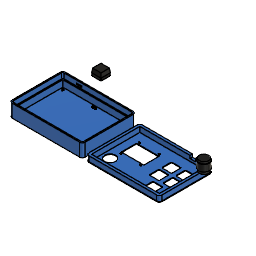
Placa (Autodesk Fusion 360 design; units mm, degrees)
Autodesk Fusion 360 part; units mm, degrees
note: some values were not read from the file. Chosen so that the rebuilt part matches the saved one: which bodies a step acts on. Set by a fixed rule: which sketch regions a step uses.
sketch "Boceto1" plane through (0, 0, 0) normal (0, 0, 1) x (1, 0, 0)
  line L0 (-2, 76) -> (102, 76)
  line L1 (106, 72) -> (106, -2)
  line L2 (102, -6) -> (-2, -6)
  line L3 (-6, -2) -> (-6, 72)
  arc A0 (102, -6) -> (106, -2) centre (102, -2) ccw
  arc A1 (106, 72) -> (102, 76) centre (102, 72) ccw
  arc A2 (-2, 76) -> (-6, 72) centre (-2, 72) ccw
  arc A3 (-6, -2) -> (-2, -6) centre (-2, -2) ccw
  line L4 (-2, 72) -> (102, 72)
  line L5 (-2, -2) -> (-2, 72)
  line L6 (102, -2) -> (-2, -2)
  line L7 (102, 72) -> (102, -2)
  line L8 (0, 0) -> (100, 0)
  line L9 (100, 0) -> (100, 70)
  line L10 (100, 70) -> (0, 70)
  line L11 (0, 70) -> (0, 0)
  circle A4 centre (1.8, 68) radius 1
  circle A5 centre (1.8, 68) radius 1.5
  circle A6 centre (1.8, 2) radius 1
  circle A7 centre (48.2, 68) radius 1
  circle A8 centre (48.2, 68) radius 1.5
  circle A9 centre (1.8, 2) radius 1.5
  circle A10 centre (48.2, 2) radius 1.5
  circle A11 centre (48.2, 2) radius 1
  circle A12 centre (98.2, 2) radius 1.5
  circle A13 centre (98.2, 2) radius 1
  circle A14 centre (51.8, 2) radius 1
  circle A15 centre (51.8, 2) radius 1.5
  circle A16 centre (51.8, 68) radius 1.5
  circle A17 centre (51.8, 68) radius 1
  circle A18 centre (98.2, 68) radius 1
  circle A19 centre (98.2, 68) radius 1.5
  arc A20 (-2, 74) -> (-4, 72) centre (-2, 72) ccw
  line L12 (-4, -2) -> (-4, 72)
  arc A21 (-4, -2) -> (-2, -4) centre (-2, -2) ccw
  line L13 (102, -4) -> (-2, -4)
  arc A22 (102, -4) -> (104, -2) centre (102, -2) ccw
  line L14 (104, 72) -> (104, -2)
  arc A23 (104, 72) -> (102, 74) centre (102, 72) ccw
  line L15 (-2, 74) -> (102, 74)
  point P0 (-6, 76)
  point P1 (106, 76)
  point P2 (-6, -6)
  point P3 (22.5, -6)
  point P4 (50, 70)
  point P5 (50, 70)
  dimension "d29" = 4
  dimension "d30" = 4
  dimension "d31" = 4
  dimension "d32" = 4
  dimension "d35" = 4
  dimension "d285" = 100
  dimension "d286" = 70
  dimension "d287" = 2
  dimension "d288" = 0.5
  dimension "d289" = 2
  dimension "d290" = 66
  dimension "d291" = 2
  dimension "d292" = 46.4
  dimension "d293" = 2
  dimension "d294" = 1.8
  dimension "d295" = 0.5
  dimension "d296" = 0.5
  dimension "d297" = 2
  dimension "d298" = 1.8
  dimension "d303" = 2
  dimension "d306" = 50
  dimension "d307" = 0
  dimension "d308" = 1.8
  dimension "d321" = 2
  dimension "d322" = 2
  dimension "d323" = -2
  constraint horizontal L0
  constraint vertical L1
  constraint horizontal L2
  constraint vertical L3
  constraint tangent L1 A0
  constraint tangent L2 A0
  constraint coincident P1 L0
  constraint coincident P1 L1
  constraint tangent L0 A1
  constraint tangent L1 A1
  constraint coincident P0 L0
  constraint coincident P0 L3
  constraint tangent L0 A2
  constraint tangent L3 A2
  constraint coincident P2 L2
  constraint coincident P2 L3
  constraint tangent L2 A3
  constraint tangent L3 A3
  constraint coincident L2 P3
  constraint horizontal L8
  constraint vertical L9
  constraint horizontal L10
  constraint vertical L11
  constraint coincident L8.start L11.end
  constraint midpoint L10 P5
  measures "d29" radius of A0
  measures "d30" radius of A1
  measures "d31" radius of A2
  measures "d32" radius of A3
  measures "d285" distance of L8.start L8.end
  measures "d286" distance of L8.start L10.end
  measures "d287" diameter of A4
  measures "d289" diameter of A6
  measures "d290" vertical distance of A4.centre A6.centre
  measures "d291" diameter of A7
  measures "d292" horizontal distance of A4.centre A7.centre
  measures "d293" distance of L10 A4.centre
  measures "d294" distance of L11 A4.centre
  measures "d297" distance of L8 A6.centre
  measures "d298" horizontal distance of A7.centre P5
  measures "d303" distance of L10 A7.centre
  measures "d308" distance of L11 A6.centre
  measures "d321" distance of L5 L11
  measures "d322" distance of L4 L10
extrude "Extruir10" add sketch "Boceto1" along normal blind 2 contours L8 L9 L10 L11 | A4 | A5 | A6 | A7 | A8 | A9 | A10 | A11 | A12 | A13 | A14 | A15 | A16 | A17 | A18 | A19 makes body 1
extrude "Extruir41" add sketch "Boceto1" along normal blind 3 separate body contours A5 makes body 2
extrude "Extruir42" add sketch "Boceto1" along normal blind 4 contours A4 bodies 2
pattern_linear "Patrón R4" count 2 spacing 66 along (0, -1, 0) count 2 spacing 46.4 along (1, 0, 0) of bodies 2 makes body 3 at (3.2981, 1.9252, 2) makes body 4 at (49.5822, 68.5827, 2) makes body 5 at (48.6063, 3.4439, 2)
pattern_linear "Patrón R5" count 2 spacing 50 along (1, 0, 0) of bodies 2 3 4 5 makes body 6 at (53.1822, 68.5827, 2) makes body 7 at (51.1157, 0.6652, 2) makes body 8 at (99.5822, 68.5827, 2) makes body 9 at (99.6981, 1.9252, 2)
combine "Combinar3" operation add target body 1 tool bodies 6 3 4 5 7 9 8 2
extrude "Extruir13" add sketch "Boceto1" along normal blind 2 contours L4 L5 L6 L7 bodies 1
extrude "Extruir14" add sketch "Boceto1" along normal blind 20 contours L0 L1 L2 L3 A0 A1 A2 A3 | A20 L12 A21 L13 A22 L14 A23 L15 bodies 1
sketch "Boceto3" plane through (0, 76, 0) normal (0, 1, 0) x (-1, 0, 0)
  line L0 (-102, 0) -> (2, 0)
  line L1 (2, 0) -> (2, 20)
  line L2 (2, 20) -> (-102, 20)
  line L3 (-102, 20) -> (-102, 0)
  line L4 (-25.1, 16) -> (-17, 16)
  line L5 (-23.55, 13) -> (-18.55, 13)
  line L6 (-25.1, 16) -> (-25.1, 14.7)
  line L7 (-17, 16) -> (-17, 14.7)
  line L8 (-17, 14.7) -> (-18.55, 13)
  line L9 (-25.1, 14.7) -> (-23.55, 13)
  line L10 (2, 0) -> (-102, 0)
  dimension "d97" = 8.1
  dimension "d98" = 5
  dimension "d99" = 3
  dimension "d101" = 1.3
  dimension "d102" = 1.3
  dimension "d103" = 19
  dimension "d105" = 16
  constraint horizontal L4
  constraint horizontal L5
  constraint perpendicular L4 L6
  constraint vertical L7
  measures "d97" distance of L4.start L4.end
  measures "d98" distance of L5.start L5.end
  measures "d99" distance of L4 L5
  measures "d101" distance of L4.start L6.end
  measures "d102" distance of L4.end L7.end
  measures "d103" distance of L1 L7
  measures "d105" distance of L4 L10
extrude "Extruir15" cut sketch "Boceto3" against normal blind 18 contours L4 L5 L6 L7 L8 L9 bodies 1
sketch "Boceto4" plane through (0, 0, 20) normal (0, 0, 1) x (-1, 0, 0)
  line L0 (2, -72) -> (-102, -72)
  line L1 (-102, -72) -> (-102, 2)
  line L2 (-102, 2) -> (2, 2)
  line L3 (2, 2) -> (2, -72)
  arc A0 (2, -76) -> (6, -72) centre (2, -72) ccw
  line L4 (6, -72) -> (6, 2)
  arc A1 (6, 2) -> (2, 6) centre (2, 2) ccw
  line L5 (2, 6) -> (-102, 6)
  arc A2 (-102, 6) -> (-106, 2) centre (-102, 2) ccw
  line L6 (-106, 2) -> (-106, -72)
  arc A3 (-106, -72) -> (-102, -76) centre (-102, -72) ccw
  line L7 (-102, -76) -> (2, -76)
  line L8 (2, 5.9687) -> (-102, 5.9687)
  arc A4 (-102, 5.9687) -> (-105.9688, 2) centre (-102, 2) ccw
  line L9 (-105.9688, 2) -> (-105.9688, -72)
  arc A5 (-105.9688, -72) -> (-102, -75.9688) centre (-102, -72) ccw
  line L10 (-102, -75.9688) -> (2, -75.9688)
  arc A6 (2, -75.9688) -> (5.9688, -72) centre (2, -72) ccw
  line L11 (5.9687, -72) -> (5.9687, 2)
  arc A7 (5.9687, 2) -> (2, 5.9688) centre (2, 2) ccw
  line L12 (2, 3.9687) -> (-102, 3.9687)
  arc A8 (-102, 3.9687) -> (-103.9688, 2) centre (-102, 2) ccw
  line L13 (-103.9688, 2) -> (-103.9688, -72)
  arc A9 (-103.9688, -72) -> (-102, -73.9688) centre (-102, -72) ccw
  line L14 (-102, -73.9688) -> (2, -73.9687)
  arc A10 (2, -73.9687) -> (3.9687, -72) centre (2, -72) ccw
  line L15 (3.9687, -72) -> (3.9688, 2)
  arc A11 (3.9688, 2) -> (2, 3.9688) centre (2, 2) ccw
  dimension "d328" = -2
extrude "Extruir16" cut sketch "Boceto4" against normal blind 8 contours L12 A8 L13 A9 L14 A10 L15 A11 bodies 1
extrude "Extruir17" add sketch "Boceto4" along normal blind 8 separate body contours L8 A4 L9 A5 L10 A6 L11 A7 | L12 A8 L13 A9 L14 A10 L15 A11 makes body 10
extrude "Extruir18" add sketch "Boceto4" along normal blind 9 contours A0 L4 A1 L5 A2 L6 A3 L7 bodies 10
extrude "Extruir19" cut sketch "Boceto4" along normal blind 8 contours A0 L4 A1 L5 A2 L6 A3 L7 bodies 10
extrude "Extruir20" add 1 faces at (32.6667, 73.3229, 28) along direction (0, 0, 1) blind 1 on bodies 10 bodies 10
extrude "Extruir21" add sketch "Boceto4" along normal blind 9 contours L0 L1 L2 L3 bodies 10
extrude "Extruir22" cut sketch "Boceto4" along normal blind 8 contours L0 L1 L2 L3 bodies 10
move_body "Desplazar1" bodies 10 to x (1, 0, 0) y (0, 1, 0) z (0, 0, 1) at (115, 0, 0)
sketch "Boceto5" plane through (0, 0, 29) normal (0, 0, 1) x (-1, 0, 0)
  line L0 (-217, -76) -> (-113, -76)
  arc A0 (-113, -76) -> (-109, -72) centre (-113, -72) ccw
  line L1 (-109, -72) -> (-109, 2)
  arc A1 (-109, 2) -> (-113, 6) centre (-113, 2) ccw
  line L2 (-113, 6) -> (-217, 6)
  arc A2 (-217, 6) -> (-221, 2) centre (-217, 2) ccw
  line L3 (-221, 2) -> (-221, -72)
  arc A3 (-221, -72) -> (-217, -76) centre (-217, -72) ccw
  line L4 (-170.1727, -59.9244) -> (-205.5227, -59.9244)
  line L5 (-205.5227, -59.9244) -> (-205.5227, -26.5744)
  line L6 (-205.5227, -26.5744) -> (-170.1727, -26.5744)
  line L7 (-170.1727, -26.5744) -> (-170.1727, -59.9244)
  circle A4 centre (-172.6727, -57.4244) radius 1.25
  line L8 (-187.8477, -59.9244) -> (-187.8477, -26.5744)
  circle A5 centre (-203.0227, -57.4244) radius 1.25
  line L9 (-170.1727, -43.2494) -> (-205.5227, -43.2494)
  circle A6 centre (-172.6727, -29.0744) radius 1.25
  circle A7 centre (-203.0227, -29.0744) radius 1.25
  line L10 (-170.6477, -54.9244) -> (-205.0477, -54.9244)
  line L11 (-205.0477, -54.9244) -> (-205.0477, -31.9244)
  line L12 (-205.0477, -31.9244) -> (-170.6477, -31.9244)
  line L13 (-170.6477, -31.9244) -> (-170.6477, -54.9244)
  circle A8 centre (-205.4274, -14.9454) radius 7.2
  circle A9 centre (-205.4274, -14.9454) radius 8.2
  line L14 (-118, -57) -> (-131, -57)
  line L15 (-132, -56) -> (-132, -43)
  line L16 (-131, -42) -> (-118, -42)
  line L17 (-117, -43) -> (-117, -56)
  arc A10 (-118, -57) -> (-117, -56) centre (-118, -56) ccw
  arc A11 (-132, -56) -> (-131, -57) centre (-131, -56) ccw
  arc A12 (-131, -42) -> (-132, -43) centre (-131, -43) ccw
  arc A13 (-117, -43) -> (-118, -42) centre (-118, -43) ccw
  arc A14 (-153.4221, -56) -> (-152.4221, -57) centre (-152.4221, -56) ccw
  line L18 (-153.4221, -56) -> (-153.4221, -43)
  arc A15 (-152.4221, -42) -> (-153.4221, -43) centre (-152.4221, -43) ccw
  line L19 (-152.4221, -42) -> (-139.4221, -42)
  arc A16 (-138.4221, -43) -> (-139.4221, -42) centre (-139.4221, -43) ccw
  line L20 (-138.4221, -43) -> (-138.4221, -56)
  arc A17 (-139.4221, -57) -> (-138.4221, -56) centre (-139.4221, -56) ccw
  line L21 (-139.4221, -57) -> (-152.4221, -57)
  arc A18 (-132.0698, -36.5317) -> (-131.0698, -37.5317) centre (-131.0698, -36.5317) ccw
  line L22 (-132.0698, -36.5317) -> (-132.0698, -23.5317)
  arc A19 (-131.0698, -22.5317) -> (-132.0698, -23.5317) centre (-131.0698, -23.5317) ccw
  line L23 (-131.0698, -22.5317) -> (-118.0698, -22.5317)
  arc A20 (-117.0698, -23.5317) -> (-118.0698, -22.5317) centre (-118.0698, -23.5317) ccw
  line L24 (-117.0698, -23.5317) -> (-117.0698, -36.5317)
  arc A21 (-118.0698, -37.5317) -> (-117.0698, -36.5317) centre (-118.0698, -36.5317) ccw
  line L25 (-118.0698, -37.5317) -> (-131.0698, -37.5317)
  arc A22 (-153.4221, -36.8108) -> (-152.4221, -37.8108) centre (-152.4221, -36.8108) ccw
  line L26 (-153.4221, -36.8108) -> (-153.4221, -23.8108)
  arc A23 (-152.4221, -22.8108) -> (-153.4221, -23.8108) centre (-152.4221, -23.8108) ccw
  line L27 (-152.4221, -22.8108) -> (-139.4221, -22.8108)
  arc A24 (-138.4221, -23.8108) -> (-139.4221, -22.8108) centre (-139.4221, -23.8108) ccw
  line L28 (-138.4221, -23.8108) -> (-138.4221, -36.8108)
  arc A25 (-139.4221, -37.8108) -> (-138.4221, -36.8108) centre (-139.4221, -36.8108) ccw
  line L29 (-139.4221, -37.8108) -> (-152.4221, -37.8108)
  arc A26 (-141.9784, -16.2261) -> (-140.9784, -17.2261) centre (-140.9784, -16.2261) ccw
  line L30 (-141.9784, -16.2261) -> (-141.9784, -3.2261)
  arc A27 (-140.9784, -2.2261) -> (-141.9784, -3.2261) centre (-140.9784, -3.2261) ccw
  line L31 (-140.9784, -2.2261) -> (-127.9784, -2.2261)
  arc A28 (-126.9784, -3.2261) -> (-127.9784, -2.2261) centre (-127.9784, -3.2261) ccw
  line L32 (-126.9784, -3.2261) -> (-126.9784, -16.2261)
  arc A29 (-127.9784, -17.2261) -> (-126.9784, -16.2261) centre (-127.9784, -16.2261) ccw
  line L33 (-127.9784, -17.2261) -> (-140.9784, -17.2261)
  point P0 (-108.3558, -46.4242)
  point P1 (-117, -57)
  point P2 (-132, -57)
  point P3 (-117, -42)
  dimension "d125" = 35.35
  dimension "d126" = 33.35
  dimension "d127" = 2.5
  dimension "d131" = 2.5
  dimension "d132" = 2.5
  dimension "d133" = 34.4
  dimension "d134" = 23
  dimension "d135" = 2.5
  dimension "d136" = 0.475
  dimension "d141" = 14.4
  dimension "d142" = 1
  dimension "d256" = 15
  dimension "d257" = 15
  dimension "d258" = 1
  dimension "d259" = 1
  dimension "d260" = 1
  dimension "d261" = 1
  dimension "d262" = 1
  constraint horizontal L4
  constraint vertical L5
  constraint horizontal L6
  constraint vertical L7
  constraint midpoint L4 L8.start
  constraint midpoint L6 L8.end
  constraint symmetric A4 L8 A5
  constraint midpoint L7 L9.start
  constraint midpoint L5 L9.end
  constraint symmetric A4 L9 A6
  constraint symmetric A5 L9 A7
  constraint horizontal L10
  constraint vertical L11
  constraint horizontal L12
  constraint vertical L13
  constraint horizontal L14
  constraint vertical L15
  constraint horizontal L16
  constraint vertical L17
  constraint coincident P1 L14
  constraint coincident P1 L17
  constraint tangent L14 A10
  constraint tangent L17 A10
  constraint coincident P2 L14
  constraint coincident P2 L15
  constraint tangent L14 A11
  constraint tangent L15 A11
  constraint equal A10 A11
  constraint tangent L15 A12
  constraint tangent L16 A12
  constraint equal A10 A12
  constraint coincident P3 L16
  constraint coincident P3 L17
  constraint tangent L16 A13
  constraint tangent L17 A13
  constraint equal A10 A13
  constraint horizontal L21
  constraint vertical L18
  constraint horizontal L19
  constraint vertical L20
  constraint tangent A17 L21
  constraint tangent L20 A17
  constraint tangent A14 L21
  constraint tangent A14 L18
  constraint equal A14 A17
  constraint tangent L18 A15
  constraint tangent A15 L19
  constraint equal A15 A17
  constraint tangent L19 A16
  constraint tangent A16 L20
  constraint equal A16 A17
  constraint horizontal L25
  constraint vertical L22
  constraint horizontal L23
  constraint vertical L24
  constraint tangent A21 L25
  constraint tangent L24 A21
  constraint tangent A18 L25
  constraint tangent A18 L22
  constraint equal A18 A21
  constraint tangent L22 A19
  constraint tangent A19 L23
  constraint equal A19 A21
  constraint tangent L23 A20
  constraint tangent A20 L24
  constraint equal A20 A21
  constraint horizontal L29
  constraint vertical L26
  constraint horizontal L27
  constraint vertical L28
  constraint tangent A25 L29
  constraint tangent L28 A25
  constraint tangent A22 L29
  constraint tangent A22 L26
  constraint equal A22 A25
  constraint tangent L26 A23
  constraint tangent A23 L27
  constraint equal A23 A25
  constraint tangent L27 A24
  constraint tangent A24 L28
  constraint equal A24 A25
  constraint horizontal L33
  constraint vertical L30
  constraint horizontal L31
  constraint vertical L32
  constraint tangent A29 L33
  constraint tangent L32 A29
  constraint tangent A26 L33
  constraint tangent A26 L30
  constraint equal A26 A29
  constraint tangent L30 A27
  constraint tangent A27 L31
  constraint equal A27 A29
  constraint tangent L31 A28
  constraint tangent A28 L32
  constraint equal A28 A29
  measures "d125" distance of L4.start L4.end
  measures "d126" distance of L4.start L6.end
  measures "d127" diameter of A4
  measures "d131" horizontal distance of L4.start A4.centre
  measures "d132" vertical distance of L4.start A4.centre
  measures "d133" distance of L10.start L10.end
  measures "d134" distance of L10.start L12.end
  measures "d135" distance of A4.centre L10
  measures "d136" distance of L5 L11
  measures "d141" diameter of A8
  measures "d256" distance of P1 P3
  measures "d257" distance of P1 P2
  measures "d258" radius of A10
  measures "d259" radius of A17
  measures "d260" radius of A21
  measures "d261" radius of A25
  measures "d262" radius of A29
extrude "Extruir23" cut sketch "Boceto5" against normal blind 5 contours L8 L9 L10 L11 | L8 L9 L10 L13 | L8 L9 L12 L13 | L8 L9 L11 L12 bodies 10
extrude "Extruir24" add sketch "Boceto5" against normal blind 2 contours A4 | A5 | A6 | A7 bodies 10
extrude "Extruir25" cut sketch "Boceto5" against normal blind 49 contours A8 | A9 bodies 10
extrude "Extruir26" add sketch "Boceto5" along normal blind 17 separate body contours A8 makes body 11
extrude "Extruir27" add sketch "Boceto5" along normal blind 14 separate body contours A9 makes body 12
extrude "Extruir28" cut sketch "Boceto5" along normal blind 4 contours A9 bodies 12
move_body "Desplazar2" bodies 11 12 to x (1, 0, 0) y (0, 1, 0) z (0, 0, 1) at (40.9619, 25.058, 2.4329)
combine "Combinar2" operation add target body 11 tool bodies 12
sketch "Boceto8" plane through (0, 0, 29) normal (0, 0, 1) x (1, 0, 0)
  arc A0 (-8.5, -7.5) -> (-7.5, -8.5) centre (-7.5, -7.5) ccw
  line L0 (-6.5, -6.5) -> (-6.5, 6.5)
  arc A1 (8.5, 7.5) -> (7.5, 8.5) centre (7.5, 7.5) ccw
  arc A2 (7.5, -8.5) -> (8.5, -7.5) centre (7.5, -7.5) ccw
  arc A3 (7.5, 6.5) -> (6.5, 7.5) centre (6.5, 6.5) ccw
  line L1 (-6.5, 6.5) -> (6.5, 6.5)
  line L2 (-7.5, -6.5) -> (-7.5, 6.5)
  line L3 (-7.5, 8.5) -> (7.5, 8.5)
  arc A4 (-6.5, 7.5) -> (-7.5, 6.5) centre (-6.5, 6.5) ccw
  line L4 (-8.5, -7.5) -> (-8.5, 7.5)
  line L5 (6.5, -7.5) -> (-6.5, -7.5)
  arc A5 (-7.5, 8.5) -> (-8.5, 7.5) centre (-7.5, 7.5) ccw
  circle A6 centre (0, 0) radius 1.5
  line L6 (-6.5, 7.5) -> (6.5, 7.5)
  line L7 (7.5, -8.5) -> (-7.5, -8.5)
  arc A7 (6.5, -7.5) -> (7.5, -6.5) centre (6.5, -6.5) ccw
  line L8 (8.5, 7.5) -> (8.5, -7.5)
  line L9 (6.5, 6.5) -> (6.5, -6.5)
  line L10 (7.5, 6.5) -> (7.5, -6.5)
  arc A8 (-7.5, -6.5) -> (-6.5, -7.5) centre (-6.5, -6.5) ccw
  line L11 (6.5, -6.5) -> (-6.5, -6.5)
  point P0 (7.5, 7.5)
  point P1 (-7.5, -7.5)
  point P2 (-7.5, 7.5)
  dimension "d241" = 1
  dimension "d242" = 15
  dimension "d243" = 15
  dimension "d244" = 1
  dimension "d245" = 1
  dimension "d246" = 1
  dimension "d247" = 1
  dimension "d248" = 1
  dimension "d249" = 1
  dimension "d250" = 1
  dimension "d251" = 1
  dimension "d252" = 1
  dimension "d253" = 7.5
  dimension "d254" = 7.5
  dimension "d255" = 3
  constraint horizontal L6
  constraint vertical L10
  constraint horizontal L5
  constraint vertical L2
  constraint tangent L4 A5
  constraint tangent L3 A5
  constraint tangent A0 L7
  constraint tangent A0 L4
  constraint equal A0 A5
  constraint tangent A2 L7
  constraint tangent A2 L8
  constraint equal A2 A5
  constraint tangent A1 L3
  constraint tangent A1 L8
  constraint equal A1 A5
  constraint coincident P2 L6
  constraint coincident P2 L2
  constraint tangent A4 L6
  constraint tangent L2 A4
  constraint coincident P0 L6
  constraint coincident P0 L10
  constraint tangent A3 L6
  constraint tangent A3 L10
  constraint tangent A7 L10
  constraint tangent L5 A7
  constraint coincident P1 L5
  constraint coincident P1 L2
  constraint tangent L5 A8
  constraint tangent L2 A8
  constraint coincident A6.centre origin
  measures "d242" distance of P0 P2
  measures "d243" distance of P1 P2
  measures "d244" distance of L5 L7
  measures "d245" distance of L2 L4
  measures "d246" distance of L3 L6
  measures "d247" distance of L8 L10
  measures "d248" radius of A5
  measures "d249" radius of A4
  measures "d250" radius of A3
  measures "d251" radius of A7
  measures "d252" radius of A8
  measures "d253" distance of A6.centre L2
  measures "d254" distance of A6.centre L6
  measures "d255" diameter of A6
extrude "Extruir32" add sketch "Boceto8" along normal blind 10 separate body contours L0 L1 L9 L11 | A6 makes body 13
extrude "Extruir34" add sketch "Boceto8" along normal blind 4 contours A3 L2 A4 L5 L6 A7 L10 A8 bodies 13
split "Dividir3" by plane through (0, 0, 33) normal (0, 0, 1) bodies 13 makes body 14 at (-2.1667, 2.1667, 39)
loft "Solevación1" add section 1 face at (-2.1667, 2.1667, 39) section 2 face at (6.8333, 2.1667, 33) on bodies 13 14 bodies 13 14
extrude "Extruir35" cut sketch "Boceto8" along normal blind 4 contours A6 bodies 13
move_body "Desplazar14" bodies 13 to x (1, 0, 0) y (0, 1, 0) z (0, 0, 1) at (38.8109, 89.6933, 0)
copy_body "CopiarPegarCuerpos4" bodies 13 makes body 15
copy_body "CopiarPegarCuerpos5" bodies 13 makes body 16
move_body "Desplazar15" bodies 16 to x (1, 0, 0) y (0, 1, 0) z (0, 0, 1) at (59, 0, 0)
move_body "Desplazar16" bodies 15 to x (1, 0, 0) y (0, 1, 0) z (0, 0, 1) at (27, 0, 0)
copy_body "CopiarPegarCuerpos6" bodies 15 13 makes body 17 makes body 18
move_body "Desplazar17" bodies 17 18 to x (1, 0, 0) y (0, 1, 0) z (0, 0, 1) at (16.8789, 23.4733, 0)
extrude "Extruir38" cut sketch "Boceto5" against normal blind 2 contours L14 L15 L16 L17 A10 A11 A12 A13 | A14 L18 A15 L19 A16 L20 A17 L21 | A18 L22 A19 L23 A20 L24 A21 L25 | A22 L26 A23 L27 A24 L28 A25 L29 | A26 L30 A27 L31 A28 L32 A29 L33 bodies 10
sketch "Boceto9" plane through (0, 75.9687, 0) normal (0, 1, 0) x (-1, 0, 0)
  line L0 (-217, 20) -> (-113, 20)
  line L1 (-113, 20) -> (-113, 28)
  line L2 (-113, 28) -> (-217, 28)
  line L3 (-217, 28) -> (-217, 20)
  line L4 (-113, 20) -> (-113, 0)
  line L5 (-140.1, 16) -> (-132, 16)
  line L6 (-138.55, 14.3) -> (-133.55, 14.3)
  line L7 (-132, 16) -> (-140.1, 16)
  line L8 (-140.1, 16) -> (-140.1, 24.2907)
  line L9 (-140.1, 24.2907) -> (-132, 24.2907)
  line L10 (-132, 24.2907) -> (-132, 16)
  line L11 (-132, 16) -> (-133.55, 14.3)
  line L12 (-140.1, 16) -> (-138.55, 14.3)
  point P0 (-113, 0)
  dimension "d266" = 5
  dimension "d267" = 1.7
  dimension "d268" = 1.55
  dimension "d270" = 19
  dimension "d271" = 16
  dimension "d272" = 20
  dimension "d273" = 8.1
  dimension "d275" = 8.2907
  constraint coincident L0.end L1.start
  constraint perpendicular L0 L4
  constraint coincident P0 L4.end
  constraint horizontal L5
  constraint horizontal L6
  constraint horizontal L7
  constraint vertical L8
  constraint horizontal L9
  constraint vertical L10
  measures "d266" distance of L6.start L6.end
  measures "d267" vertical distance of L5.start L6.start
  measures "d268" horizontal distance of L5.start L6.start
  measures "d270" distance of L4 L5.end
  measures "d271" vertical distance of P0 L5.start
  measures "d272" distance of L0.end P0
  measures "d273" distance of L8.end L9.end
  measures "d275" distance of L5.end L9.end
extrude "Extruir39" cut sketch "Boceto9" against normal blind 2 contours L0 L8 L9 L10 | L0 L5 L7 L8 L10 | L5 L6 L7 L11 L12 bodies 10
extrude "Extruir40" cut sketch "Boceto9" against normal blind 4 contours L0 L8 L9 L10 | L0 L5 L7 L8 L10 | L5 L6 L7 L11 L12 bodies 10
move_body "Desplazar19" bodies 10 to x (-1, 0, 0) y (0, 1, 0) z (0, 0, -1) at (333, 0, 29)
hidden bodies 15 16 17 18
equation "d23 = 50.00 mm"
equation "d103 = 14 mm + 3 mm + 2 mm"
equation "d136 = ( ( 35.35 - 34.4 ) / 2 ) * 1 mm"
equation "d242 = d243"
equation "d253 = d254"
equation "d254 = d242 / 2"
equation "d256 = d243"
equation "d257 = d243"
equation "d258 = d248"
equation "d259 = d248"
equation "d260 = d248"
equation "d261 = d248"
equation "d262 = d248"
equation "d266 = d98"
equation "d267 = d99 - d101"
equation "d268 = ( d97 - d98 ) / 2"
equation "d270 = d103"
equation "d271 = d105"
equation "d273 = d97"
equation "d282 = d23"
equation "d289 = d287"
equation "d291 = d287"
equation "d293 = ( d286 - d290 ) / 2"
equation "d294 = ( d285 / 2 - d292 ) / 2"
equation "d295 = d288"
equation "d296 = d288"
equation "d303 = d293"
equation "d308 = d294"
equation "d315 = d290"
equation "d316 = -d292"
equation "d323 = -d35 / 2"
equation "d328 = d323"
named bodies: "Base", "Tapa", "Encoder", "Tecla", "Tecla (2)", "Tecla (2) (1)", "Tecla (3)", "Tecla (2) (1) (1)", "Tecla (2) (2)", "Tecla (4)", "Tecla (1)"
